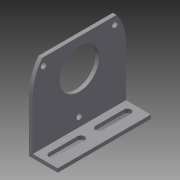
# Autodesk Inventor part: CIM Bracket
Saved by Autodesk Inventor 2015 (Build 190159000, 159)
## iProperties
Created: 2015-01-29
Part Number: CIM Bracket
Material: Generic
Document SubType Name: Modeling
Designer: pltwe4
Density: 1 g/cm^3
Appearance: Default
Author: pltwe4
Autodesk Inventor part; units mm, degrees
ref_plane "YZ Plane" through (0, 0, 0) normal (1, 0, 0) x (0, 1, 0)
ref_plane "XZ Plane" through (0, 0, 0) normal (0, 1, 0) x (-1, 0, 0)
ref_plane "XY Plane" through (0, 0, 0) normal (0, 0, 1) x (1, 0, 0)
sketch "Sketch2" plane through (0, 0, 0) normal (0, 1, 0) x (-1, 0, 0)
  line L0 (38.1, 25.4) -> (-38.1, 25.4)
  line L1 (-38.1, 25.4) -> (-38.1, -25.4)
  line L2 (-38.1, -25.4) -> (38.1, -25.4)
  line L3 (38.1, -25.4) -> (38.1, 25.4)
  line L4 (34.798, 22.098) -> (-34.798, 22.098)
  line L5 (-34.798, 22.098) -> (-34.798, -22.098)
  line L6 (-34.798, -22.098) -> (34.798, -22.098)
  line L7 (34.798, -22.098) -> (34.798, 22.098)
  line L8 (0, -35.56) -> (0, 35.56) projected
  line L9 (-53.34, 0) -> (53.34, 0) projected
  point P0 (0, 0)
  dimension "d0" = 3.302
  dimension "d1" = 76.2
  dimension "d2" = 50.8
  constraints: 16 end point, 4 parallel, 2 perpendicular, 1 horizontal, 5 other
  measures "d0" distance between parallel lines of L7 L3
  measures "d1" distance between parallel lines of L1 L3
  measures "d2" distance between parallel lines of L0 L2
extrude "Extrusion1" add sketch "Sketch2" along normal mid plane 82.55 contours L3 L9 L7 L4 L8 L0 | L8 L4 L5 L9 L1 L0 | L3 L2 L8 L6 L7 L9 | L9 L5 L6 L8 L2 L1
sketch "Sketch4" plane through (-34.798, -41.275, -22.098) normal (0, 0, 1) x (1, 0, 0)
  line L0 (0, 0) -> (0, 82.55) projected
  line L1 (69.596, 0) -> (0, 0) projected
  line L2 (69.596, 0) -> (69.596, 82.55) projected
  line L3 (0, 82.55) -> (69.596, 82.55) projected
  arc A0 (0, 8.3506) -> (0, 74.1994) centre (24.892, 41.275) ccw
  line L4 (-18.542, 41.275) -> (88.138, 41.275) projected
  line L5 (0, 8.3506) -> (0, 74.1994)
  line L6 (72.898, 82.55) -> (-3.302, 82.55) construction
  circle A1 centre (24.892, 41.275) radius 17.526
  line L7 (-3.302, 0) -> (72.898, 0) projected
  line L8 (24.892, 0) -> (-3.302, 0)
  line L9 (-3.302, 0) -> (-3.302, 82.55)
  line L10 (-3.302, 0) -> (-3.302, 82.55) projected
  line L11 (-3.302, 82.55) -> (24.892, 82.55)
  circle A2 centre (61.4172, 41.275) radius 2.54
  circle A3 centre (6.6294, 72.9068) radius 2.54
  circle A4 centre (6.6294, 9.6432) radius 2.54
  point P0 (34.798, 41.275)
  dimension "d9" = 44.704
  dimension "d13" = 35.052
  dimension "d26" = 36.5252
  dimension "d27" = 5.08
  dimension "d30" = 360
  constraints: 8 end point, 5 centre point, 4 point on circle, 3 collinear, 3 point on line, 3 tangent, 1 coincident, 1 perpendicular, 1 vertical, 7 other
  measures "d9" distance from line of L2 A0.centre
  measures "d13" diameter of A1
  measures "d26" distance of A2.centre A0.centre
  measures "d27" diameter of A2
extrude "Extrusion3" cut sketch "Sketch4" along normal up to surface (47.498 mm away) contours L7 L9 L4 L0 | L0 A0 L1 | L4 L9 L11 L0 | L0 L3 A0 | A1 L4 | L4 A1 | A2 L4 | L4 A2 | A3 | A4
extrude "Extrusion4" cut sketch "Sketch4" against normal up to surface (3.302 mm away) contours L7 L9 L4 L0 | L0 A0 L1 | L4 L9 L11 L0 | L0 L3 A0 | A1 L4 | L4 A1 | A2 L4 | L4 A2 | A3 | A4
sketch "Sketch5" plane through (38.1, -41.275, -25.4) normal (1, 0, 0) x (0, 0, -1)
  line L0 (0, 0) -> (0, 82.55) projected
  line L1 (-50.8, 82.55) -> (0, 82.55) projected
  line L2 (-50.8, 0) -> (-50.8, 82.55) projected
  line L3 (0, 0) -> (-50.8, 0) projected
  line L4 (-25.4, 0) -> (-25.4, 82.55)
  line L5 (-50.8, 82.55) -> (0, 82.55) projected
  point P0 (-25.4, 41.275)
  dimension "d18" = 25.4
  constraints: 2 end point, 2 midpoint, 1 perpendicular
  measures "d18" distance between parallel lines of L0 L4
extrude "Extrusion5" cut sketch "Sketch5" against normal up to surface (72.898 mm away) contours L3 L2 L1 L4
sketch "Sketch6" plane through (34.798, -41.275, -22.098) normal (-1, 0, 0) x (0, 0, 1)
  line L0 (22.098, 0) -> (22.098, 82.55) projected
  line L1 (0, 0) -> (0, 82.55) projected
  line L2 (44.196, 0) -> (0, 0) projected
  arc A0 (12.573, 74.6125) -> (6.223, 74.6125) centre (9.398, 74.6125) ccw
  arc A1 (6.223, 7.9375) -> (12.573, 7.9375) centre (9.398, 7.9375) ccw
  arc A2 (6.223, 49.2125) -> (12.573, 49.2125) centre (9.398, 49.2125) ccw
  arc A3 (12.573, 33.3375) -> (6.223, 33.3375) centre (9.398, 33.3375) ccw
  line L3 (12.573, 33.3375) -> (12.573, 7.9375)
  line L4 (6.223, 7.9375) -> (6.223, 33.3375)
  line L5 (12.573, 49.2125) -> (12.573, 74.6125)
  line L6 (6.223, 74.6125) -> (6.223, 49.2125)
  line L7 (22.098, 41.275) -> (0, 41.275) construction
  line L8 (6.223, 61.9125) -> (12.573, 61.9125) construction
  line L9 (0, 82.55) -> (22.098, 82.55) construction
  line L10 (0, 82.55) -> (44.196, 82.55) construction
  line L11 (9.398, 74.6125) -> (9.398, 49.2125) construction
  point P0 (22.098, 41.275)
  dimension "d21" = 6.35
  dimension "d22" = 25.4
  dimension "d23" = 12.7
  constraints: 16 end point, 8 point on circle, 8 tangent, 4 centre point, 4 midpoint, 2 parallel, 1 collinear, 1 equal radius, 1 vertical, 5 other
  measures "d21" diameter of A0
  measures "d22" distance of L11.start L11.end
  measures "d23" distance between parallel lines of L0 L11
extrude "Extrusion6" cut sketch "Sketch6" against normal up to next
equation "\"d0\" = WallThickness"
equation "\"d3\" = DiameterMotor"
equation "\"d13\" = InnerHole"
equation "\"d26\" = Distance2Screw"
equation "\"WallThickness\" = 3.302"
equation "\"DiameterMotor\" = 82.55"
equation "\"InnerHole\" = 35.052"
equation "\"Distance2Screw\" = 36.5252"
equation "\"ScrewDiameter\" = 5.08"
body "Solid1"
